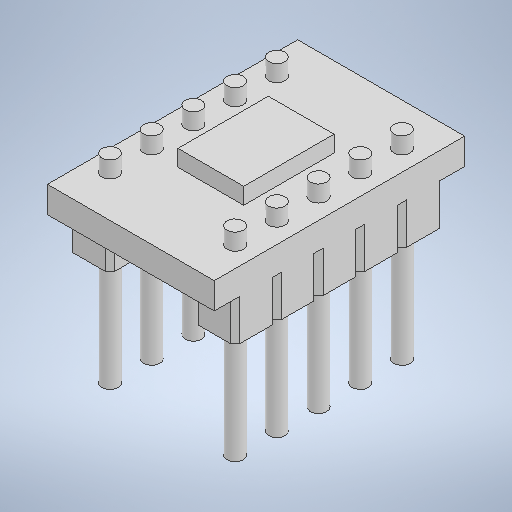
# Autodesk Inventor part: bno055_module
Saved by Autodesk Inventor 2025 (Build 290162000, 162)
## iProperties
Created: 2024-08-31
Part Number: bno055_module
Material: 一般
Document SubType Name: Modeling
Designer: 8326d
Density: 1 g/cm^3
Appearance: 既定
Author: 8326d
Autodesk Inventor part; units mm, degrees
ref_plane "YZ Plane" through (0, 0, 0) normal (1, 0, 0) x (0, 1, 0)
ref_plane "XZ Plane" through (0, 0, 0) normal (0, 1, 0) x (-1, 0, 0)
ref_plane "XY Plane" through (0, 0, 0) normal (0, 0, 1) x (1, 0, 0)
sketch "スケッチ1" plane through (0, 0, 0) normal (0, 1, 0) x (-1, 0, 0)
  line L0 (-5.08, 7.62) -> (5.08, 7.62)
  line L1 (5.08, 7.62) -> (5.08, -7.62)
  line L2 (5.08, -7.62) -> (-5.08, -7.62)
  line L3 (-5.08, -7.62) -> (-5.08, 7.62)
  line L4 (-5.08, 7.62) -> (5.08, -7.62) construction
  line L5 (5.08, 7.62) -> (-5.08, -7.62) construction
  point P0 (0, 0)
  dimension "d0" = 10.16
  dimension "d1" = 15.24
  constraints: 12 end point, 2 midpoint, 2 parallel, 1 horizontal, 1 perpendicular
  measures "d0" distance of L1.end L2.end
  measures "d1" distance of L0.end L1.end
extrude "押し出し1" add sketch "スケッチ1" along normal blind 1.6
sketch "スケッチ2" plane through (0, 1.6, 0) normal (0, 1, 0) x (1, 0, 0)
  line L0 (2, -2.75) -> (-2, -2.75)
  line L1 (-2, -2.75) -> (-2, 2.75)
  line L2 (-2, 2.75) -> (2, 2.75)
  line L3 (2, 2.75) -> (2, -2.75)
  line L4 (2, -2.75) -> (-2, 2.75) construction
  line L5 (-2, -2.75) -> (2, 2.75) construction
  point P0 (0, 0)
  dimension "d4" = 4
  dimension "d5" = 5.5
  constraints: 12 end point, 2 midpoint, 2 parallel, 1 horizontal, 1 perpendicular
  measures "d4" distance of L1.end L2.end
  measures "d5" distance of L0.end L1.end
extrude "押し出し2" add sketch "スケッチ2" along normal blind 1
sketch "スケッチ3" plane through (0, 0, 0) normal (0, -1, 0) x (1, 0, 0)
  line L0 (2.54, 6.35) -> (5.08, 6.35)
  line L1 (5.08, 6.35) -> (5.08, 3.81)
  line L2 (5.08, 3.81) -> (2.54, 3.81)
  line L3 (2.54, 3.81) -> (2.54, 6.35)
  line L4 (2.54, 6.35) -> (5.08, 3.81) construction
  line L5 (5.08, 6.35) -> (2.54, 3.81) construction
  line L6 (1.5528, 5.08) -> (3.81, 2.8228)
  line L7 (3.81, 2.8228) -> (6.0672, 5.08)
  line L8 (6.0672, 5.08) -> (3.81, 7.3372)
  line L9 (3.81, 7.3372) -> (1.5528, 5.08)
  line L10 (1.5528, 5.08) -> (6.0672, 5.08) construction
  line L11 (3.81, 2.8228) -> (3.81, 7.3372) construction
  point P0 (0, 0)
  point P1 (3.81, 5.08)
  point P2 (3.81, 5.08)
  point P3 (3.81, 5.08)
  point P4 (2.8228, 6.35)
  point P5 (2.54, 6.0672)
  point P6 (2.54, 4.0928)
  point P7 (2.8228, 3.81)
  point P8 (4.7972, 3.81)
  point P9 (5.08, 4.0928)
  point P10 (5.08, 6.0672)
  point P11 (4.7972, 6.35)
  dimension "d8" = 2.54
  dimension "d9" = 2.54
  dimension "d10" = 5.08
  dimension "d11" = 3.81
  dimension "d31" = 0.2
  constraints: 24 end point, 6 midpoint, 4 parallel, 2 perpendicular, 1 horizontal, 1 horizontal alignment, 1 vertical alignment
  measures "d8" distance of L1.end L2.end
  measures "d9" distance of L0.end L1.end
  measures "d10" vertical distance of point (0, 0) point (3.81, 5.08)
  measures "d11" horizontal distance of point (0, 0) point (3.81, 5.08)
  measures "d31" distance from line of L0.end L8
extrude "押し出し3" add sketch "スケッチ3" along normal blind 2.5 contours L0 L8 L1 L7 L2 L6 L3 L9
sketch "スケッチ4" plane through (0, -2.5, 0) normal (0, -1, 0) x (1, 0, 0)
  line L0 (4.7972, 6.35) -> (2.8228, 6.35) projected
  line L1 (5.08, 4.0928) -> (5.08, 6.0672) projected
  circle A0 centre (3.81, 5.08) radius 0.5
  point P0 (0, 0)
  point P1 (4.88, 6.35)
  point P2 (2.74, 6.35)
  point P3 (5.08, 4.01)
  point P4 (5.08, 6.15)
  point P5 (5.08, 5.08)
  point P6 (3.81, 6.35)
  point P7 (5.08, 6.35)
  point P8 (2.54, 6.35)
  point P9 (5.08, 3.81)
  dimension "d17" = 1
  constraints: 2 midpoint, 1 centre point, 1 horizontal alignment, 1 vertical alignment
  measures "d17" diameter of A0
extrude "押し出し4" add sketch "スケッチ4" along normal blind 7
sketch "スケッチ5" plane through (0, 1.6, 0) normal (0, 1, 0) x (1, 0, 0)
  circle A0 centre (3.81, -5.08) radius 0.5 projected
  circle A1 centre (3.81, -5.08) radius 0.5 projected
  point P0 (0, 0)
extrude "押し出し5" add sketch "スケッチ5" along normal blind 1
pattern_linear "矩形状パターン2" count 5 spacing 2.54 along (0, 0, -1) count 2 spacing 7.62 along (-1, 0, 0) of "押し出し3", "押し出し4", "押し出し5"
